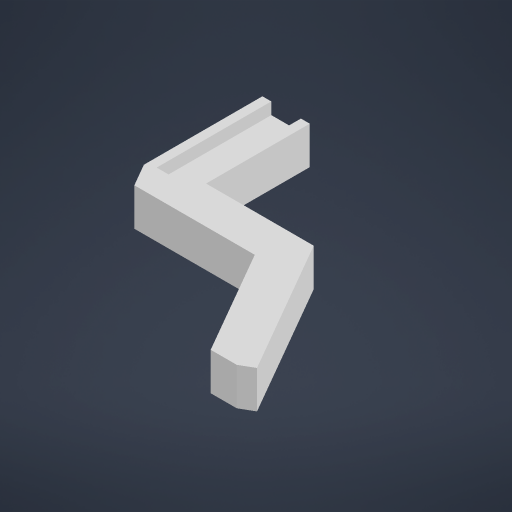
# Autodesk Inventor part: HorizGrabberMoving
Saved by Autodesk Inventor 2024.2 (Build 282272000, 272)
## iProperties
Created: 2024-02-28
Part Number: HorizGrabberMoving
Material: Generic
Document SubType Name: Modeling
Designer: Jared
Density: 1 g/cm^3
Appearance: Default
Author: Jared
Autodesk Inventor part; units mm, degrees
ref_plane "YZ Plane" through (0, 0, 0) normal (1, 0, 0) x (0, 1, 0)
ref_plane "XZ Plane" through (0, 0, 0) normal (0, 1, 0) x (-1, 0, 0)
ref_plane "XY Plane" through (0, 0, 0) normal (0, 0, 1) x (1, 0, 0)
ref_plane "Work Plane1" through (0, 12.7, 0) normal (0, 1, 0) x (1, 0, 0)
sketch "Sketch3" plane through (0, 12.7, 0) normal (0, 1, 0) x (1, 0, 0)
  line L0 (-144.4503, 24.8067) -> (-122.2253, 63.3015)
  line L1 (-126.6247, 70.9215) -> (-122.2253, 63.3015)
  line L2 (-122.2253, 63.3015) -> (-81.5853, 63.3015)
  line L3 (-126.6247, 70.9215) -> (-151.3441, 28.1063)
  line L4 (-133.3378, 44.0541) -> (-139.9369, 47.8641)
  line L5 (-151.3441, 28.1063) -> (-142.5453, 28.1063)
  line L6 (-126.6247, 70.9215) -> (-77.1859, 70.9215)
  line L7 (-81.5853, 63.3015) -> (-77.1859, 70.9215)
  line L8 (-151.3441, 28.1063) -> (-155.6743, 30.6063)
  line L9 (-151.3441, 28.1063) -> (-146.3441, 28.1063) construction
  line L10 (-155.6743, 30.6063) -> (-129.5115, 75.9215)
  line L11 (-130.9549, 73.4215) -> (-126.6247, 70.9215)
  line L12 (-126.6247, 70.9215) -> (-129.5115, 75.9215)
  line L13 (-126.6247, 70.9215) -> (-119.7825, 70.9215) construction
  line L14 (-80.0727, 75.9215) -> (-77.1859, 70.9215)
  line L15 (-129.5115, 75.9215) -> (-80.0727, 75.9215)
  line L16 (-91.4611, 75.9215) -> (-90.9796, 70.9215)
  point P0 (-77.3883, 70.9215)
  dimension "d84" = 44.45
  dimension "d85" = 120
  dimension "d86" = 7.62
  dimension "d105" = 120
  dimension "d133" = 40.64
  dimension "d134" = 120
  dimension "d135" = 7.62
  dimension "d160" = 90
  dimension "d163" = 5
  dimension "d164" = 150
  dimension "d166" = 5
  dimension "d168" = 120
  constraints: 34 end point, 6 point on line, 5 horizontal, 3 equal length, 1 midpoint, 1 perpendicular, 1 other
  measures "d84" distance of L0.start L1.end
  measures "d85" angle of L1 L0
  measures "d86" distance of L4.start L4.end
  measures "d105" angle of L0 L2
  measures "d133" distance of L1.end L2.end
  measures "d134" angle of L7 L2
  measures "d135" distance between parallel lines of L6 L2
  measures "d160" angle of L3 L4
  measures "d163" distance of L3.end L8.end
  measures "d164" angle of L9 L8
  measures "d166" distance of L11.start L1.start
  measures "d168" angle of L13 L12
ref_plane "Work Plane2" through (0, 88.9, 0) normal (0, 1, 0) x (1, 0, 0)
extrude "Extrusion16" add sketch "Sketch3" along normal blind 12.7 contours L5 L3 L4 L0 | L4 L3 L1 L0 | L1 L6 L7 L2
sketch "Sketch8" plane through (0, 12.7, 0) normal (0, -1, 0) x (1, 0, 0)
  line L0 (-81.5853, -63.3015) -> (-77.1859, -70.9215) projected
  line L1 (-77.1859, -70.9215) -> (-73.0826, -70.9215) construction
  line L2 (-77.1859, -70.9215) -> (-77.1859, -110.9215)
  line L3 (-77.1859, -70.9215) -> (-126.6247, -70.9215) projected
  line L4 (-77.1859, -70.9215) -> (-37.1859, -70.9215) construction
  line L5 (-77.1859, -110.9215) -> (-93.1859, -110.9215)
  line L6 (-93.1859, -110.9215) -> (-93.1859, -70.9215)
  point P0 (0, 0)
  dimension "d137" = 40
  dimension "d138" = 90
  dimension "d139" = 16
  constraints: 10 end point, 3 horizontal, 3 perpendicular, 1 point on line
  measures "d137" distance of L0.end L2.end
  measures "d138" angle of L2 L4
  measures "d139" distance of L2.end L5.end
extrude "Extrusion18" add sketch "Sketch8" against normal blind 12.7
sketch "Sketch9" plane through (0, 25.4, 0) normal (0, 1, 0) x (1, 0, 0)
  line L0 (-93.1859, 110.9215) -> (-77.1859, 110.9215) projected
  line L1 (-77.1859, 110.9215) -> (-80.1859, 110.9215)
  line L2 (-93.1859, 110.9215) -> (-90.1859, 110.9215)
  line L3 (-80.1859, 110.9215) -> (-80.1859, 72.2521)
  line L4 (-80.1859, 110.9215) -> (-41.5165, 110.9215) construction
  line L5 (-90.1859, 110.9215) -> (-90.1859, 72.2521)
  line L6 (-90.1859, 72.2521) -> (-80.1859, 72.2521)
  point P0 (0, 0)
  dimension "d142" = 3
  dimension "d143" = 3
  dimension "d144" = 90
  constraints: 12 end point, 2 perpendicular, 2 point on line, 1 horizontal, 1 vertical
  measures "d142" distance of L0.end L1.end
  measures "d143" distance of L0.start L2.end
  measures "d144" angle of L3 L4
extrude "Extrusion20" [suppressed]
extrude "Extrusion21" cut sketch "Sketch9" against normal blind 4
extrude "Extrusion22" add sketch "Sketch3" along normal blind 12.7 contours L8 L10 L11 L3 | L12 L15 L16 L6 | L11 L10 L12
mirror "Mirror1" about plane through (0, 0, 0) normal (1, 0, 0) remove original yes
body "Solid7"
